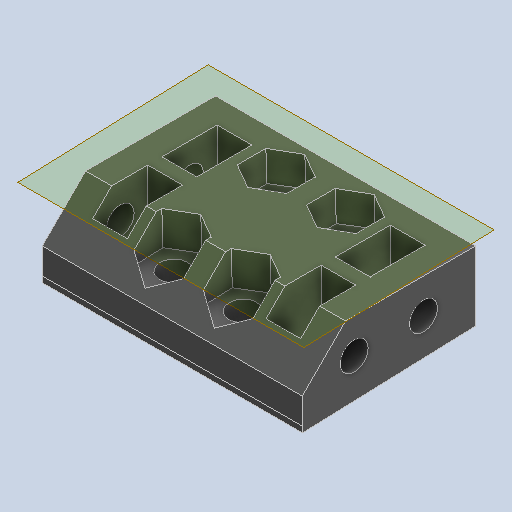
# Autodesk Inventor part: fork_middle
Saved by Autodesk Inventor 2024.1 (Build 281209000, 209)
## iProperties
Created: 2025-01-18
Part Number: fork_middle
Material: 一般
Document SubType Name: Modeling
Designer: hibik
Density: 1 g/cm^3
Appearance: 既定
Author: hibik
Autodesk Inventor part; units mm, degrees
ref_plane "YZ Plane" through (0, 0, 0) normal (1, 0, 0) x (0, 1, 0)
ref_plane "XZ Plane" through (0, 0, 0) normal (0, 1, 0) x (-1, 0, 0)
ref_plane "XY Plane" through (0, 0, 0) normal (0, 0, 1) x (1, 0, 0)
sketch "スケッチ1" plane through (0, 0, 0) normal (1, 0, 0) x (0, 1, 0)
  line L0 (4, 0) -> (-4, 0)
  line L1 (-4, 0) -> (-4, 22)
  line L2 (-4, 22) -> (4, 22)
  line L3 (4, 22) -> (4, 0)
  line L4 (4, 2) -> (-4, 2)
  point P0 (0, 0)
  point P1 (0, 0)
  dimension "d0" = 8
  dimension "d1" = 22
  dimension "d14" = 2
  constraints: 10 end point, 2 horizontal, 2 parallel, 2 point on line, 1 coincident, 1 midpoint, 1 perpendicular
  measures "d0" distance of L1.end L2.end
  measures "d1" distance of L2.end L0.start
  measures "d14" distance between parallel lines of L0 L4
extrude "押し出し1" add sketch "スケッチ1" along normal blind 15 contours L4 L1 L2 L3
sketch "スケッチ2" plane through (15, 0, 0) normal (1, 0, 0) x (0, 0, -1)
  circle A0 centre (-8, 0) radius 1.6
  circle A1 centre (-16, 0) radius 1.6
  point P0 (0, 0)
  dimension "d4" = 3.2
  dimension "d5" = 3.2
  dimension "d7" = 8
  dimension "d16" = 8
  constraints: 2 centre point, 2 horizontal alignment
  measures "d4" diameter of A0
  measures "d5" diameter of A1
  measures "d7" distance of A0.centre A1.centre
  measures "d16" distance of point (0, 0) A0.centre
extrude "押し出し2" cut sketch "スケッチ2" against normal blind 3
sketch "スケッチ3" plane through (12, 0, 8) normal (1, 0, 0) x (0, 0, -1)
  line L0 (-1.5877, -2.75) -> (-3.1754, 0)
  line L1 (-3.1754, 0) -> (-1.5877, 2.75)
  line L2 (-1.5877, 2.75) -> (1.5877, 2.75)
  line L3 (1.5877, 2.75) -> (3.1754, 0)
  line L4 (3.1754, 0) -> (1.5877, -2.75)
  line L5 (1.5877, -2.75) -> (-1.5877, -2.75)
  circle A0 centre (0, 0) radius 1.6 projected
  circle A1 centre (-8, 0) radius 1.6 projected
  line L6 (-9.5877, -2.75) -> (-11.1754, 0)
  line L7 (-11.1754, 0) -> (-9.5877, 2.75)
  line L8 (-9.5877, 2.75) -> (-6.4123, 2.75)
  line L9 (-6.4123, 2.75) -> (-4.8246, 0)
  line L10 (-4.8246, 0) -> (-6.4123, -2.75)
  line L11 (-6.4123, -2.75) -> (-9.5877, -2.75)
  line L12 (-17, 0) -> (-17, 4)
  line L13 (6, 4) -> (-14, 4) projected
  line L14 (-4.8246, 0) -> (-4.8246, 4)
  line L15 (-3.1754, 0) -> (-3.1754, 4)
  line L16 (3.1754, 0) -> (3.1754, 4)
  circle A2 centre (0, 0) radius 1.6 projected
  circle A3 centre (-8, 0) radius 1.6 projected
  line L17 (-14, 4) -> (-14, -4) projected
  line L18 (-14, -4) -> (6, -4) projected
  line L19 (6, 4) -> (-14, 4) projected
  line L20 (-11.1754, 0) -> (-11.1754, 4)
  line L21 (6, -4) -> (6, 4) projected
  point P0 (8, 0)
  point P1 (8, 4)
  point P2 (-9, 0.3038)
  point P3 (-9, 0.3038)
  point P4 (-9, -0.3038)
  point P5 (-3, -0.3038)
  point P6 (-3, 0.3038)
  point P7 (-3.6184, 1.375)
  point P8 (-2.8246, 0)
  point P9 (-2.8246, 0.6077)
  point P10 (-9, 1.249)
  point P11 (-9, -1.249)
  point P12 (-9, 2.75)
  dimension "d11" = 5.5
  constraints: 34 end point, 5 point on line, 3 parallel, 2 coincident, 2 horizontal, 1 collinear, 1 perpendicular, 1 vertical, 26 other
  measures "d11" distance between parallel lines of L11 L8
extrude "押し出し3" cut sketch "スケッチ3" against normal blind 4 contours L0 L1 L2 L3 L4 L5 | L15 L13 L16 L3 L2 L1 | L14 L9 L8 L7 L20 L13 | L10 L11 L6 L7 L8 L9 | A0 | A1
mirror "ミラー1" about plane through (0, 0, 12) normal (-1, 0, 0)
sketch "スケッチ7" plane through (15, 0, 0) normal (1, 0, 0) x (0, 0, -1)
  line L0 (-22, -4) -> (-2, -4) projected
  line L1 (-22, -4) -> (-21.9756, -4.6976)
  line L2 (-21.9756, -4.6976) -> (-2, -4)
  point P0 (0, 0)
  dimension "d22" = 2
  constraints: 4 end point, 1 perpendicular
  measures "d22" angle of L0 L2
extrude "押し出し6" add sketch "スケッチ7" against normal up to surface (30 mm away)
sketch "スケッチ8" plane through (-15, -4, 2) normal (0, -0.9993908, -0.0348995) x (1, 0, 0)
  circle A0 centre (19, 15.7147) radius 1.6
  circle A1 centre (11, 15.7147) radius 1.6
  circle A2 centre (19, 3.7147) radius 1.6
  circle A3 centre (11, 3.7147) radius 1.6
  line L0 (30, 19.9878) -> (0, 19.9878) construction
  line L1 (0, -0.2792) -> (30, -0.2792) construction
  line L2 (15, 19.9878) -> (15, -0.2792) construction
  line L3 (30, -0.2792) -> (30, 19.7086) construction
  line L4 (30, 9.7147) -> (0, 9.7147) construction
  line L5 (0, -0.2792) -> (0, 19.7086) construction
  point P0 (15, -2.1384)
  dimension "d25" = 3.2
  dimension "d26" = 8
  dimension "d27" = 12
  constraints: 4 centre point, 4 end point, 4 midpoint, 3 equal radius, 3 symmetric about line, 1 coincident
  measures "d25" diameter of A0
  measures "d26" distance of point (11, 3.715) A2.centre
  measures "d27" distance of A0.centre A2.centre
extrude "押し出し7" cut sketch "スケッチ8" against normal through all
chamfer "面取り1" distance 5 angle 45 1 edges at (0, 4, 22)
ref_plane "作業平面1" through (-15, 5.9939, 2.349) normal (0, -0.9993908, -0.0348995) x (1, 0, 0)
sketch "スケッチ10" plane through (-15, 5.9939, 2.349) normal (0, -0.9993908, -0.0348995) x (1, 0, 0)
  circle A0 centre (11, 3.7147) radius 1.6 projected
  circle A1 centre (19, 3.7147) radius 1.6 projected
  circle A2 centre (11, 15.7147) radius 1.6 projected
  circle A3 centre (19, 15.7147) radius 1.6 projected
  line L0 (0, 19.9878) -> (0, 0) projected
  line L1 (0, 0) -> (30, 0) projected
  line L2 (30, 19.9878) -> (30, 0) projected
  line L3 (30, 19.9878) -> (0, 19.9878) projected
  line L4 (11, 19.0056) -> (13.85, 17.3602)
  line L5 (13.85, 17.3602) -> (13.85, 14.0693)
  line L6 (13.85, 14.0693) -> (11, 12.4238)
  line L7 (11, 12.4238) -> (8.15, 14.0693)
  line L8 (8.15, 14.0693) -> (8.15, 17.3602)
  line L9 (8.15, 17.3602) -> (11, 19.0056)
  line L10 (11, 7.0056) -> (13.85, 5.3602)
  line L11 (13.85, 5.3602) -> (13.85, 2.0693)
  line L12 (13.85, 2.0693) -> (11, 0.4238)
  line L13 (11, 0.4238) -> (8.15, 2.0693)
  line L14 (8.15, 2.0693) -> (8.15, 5.3602)
  line L15 (8.15, 5.3602) -> (11, 7.0056)
  line L16 (21.85, 17.3602) -> (21.85, 14.0693)
  line L17 (21.85, 14.0693) -> (19, 12.4238)
  line L18 (19, 12.4238) -> (16.15, 14.0693)
  line L19 (16.15, 14.0693) -> (16.15, 17.3602)
  line L20 (16.15, 17.3602) -> (19, 19.0056)
  line L21 (19, 19.0056) -> (21.85, 17.3602)
  line L22 (21.85, 5.3602) -> (21.85, 2.0693)
  line L23 (21.85, 2.0693) -> (19, 0.4238)
  line L24 (19, 0.4238) -> (16.15, 2.0693)
  line L25 (16.15, 2.0693) -> (16.15, 5.3602)
  line L26 (16.15, 5.3602) -> (19, 7.0056)
  line L27 (19, 7.0056) -> (21.85, 5.3602)
  point P0 (15, -2.1384)
  dimension "d34" = 5.7
  constraints: 48 end point, 4 coincident, 4 vertical, 3 equal length, 52 other
  measures "d34" distance between parallel lines of L5 L8
extrude "押し出し8" cut sketch "スケッチ10" along normal blind 5.5 contours A0 | A1 | A2 | A3 | L4 L5 L6 L7 L8 L9 | L10 L11 L12 L13 L14 L15 | L16 L17 L18 L19 L20 L21 | L22 L23 L24 L25 L26 L27
